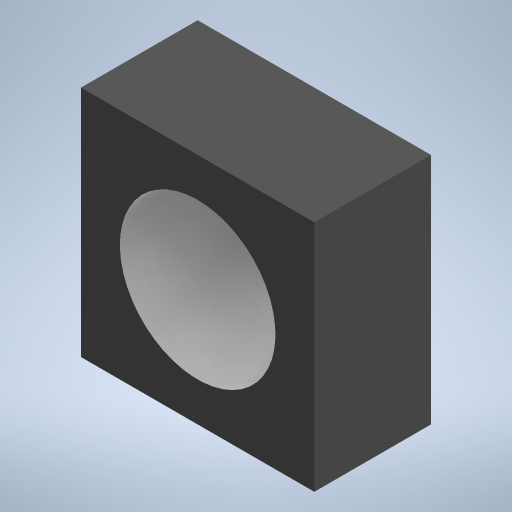
# Autodesk Inventor part: inge
Saved by Autodesk Inventor 2023.2 (Build 272271030, 271C)
## iProperties
Created: 2023-07-19
Part Number: inge
Material: Generic
Document SubType Name: Modeling
Designer: Cris Pat
Density: 1 g/cm^3
Appearance: Generic
Author: Cris Pat
Autodesk Inventor part; units mm, degrees
ref_plane "YZ Plane" through (0, 0, 0) normal (1, 0, 0) x (0, 1, 0)
ref_plane "XZ Plane" through (0, 0, 0) normal (0, 1, 0) x (-1, 0, 0)
ref_plane "XY Plane" through (0, 0, 0) normal (0, 0, 1) x (1, 0, 0)
sketch "Sketch1" plane through (0, 0, 0) normal (0, 0, 1) x (1, 0, 0)
  arc A0 (0, 50) -> (0, -50) centre (0, 0) ccw
  line L0 (0, -70) -> (0, 70) projected
  dimension "d0" = 100
  constraints: 2 point on circle, 2 point on line, 1 centre point, 1 coincident
  measures "d0" diameter of A0
revolve "Revolution1" add sketch "Sketch1" angle 360 about axis through (0, -10, 0) along (0, 1, 0)
sketch "Sketch2" plane through (0, 0, 0) normal (0, 0, 1) x (1, 0, 0)
  line L0 (-75, -75) -> (75, -75)
  line L1 (75, -75) -> (75, 75)
  line L2 (75, 75) -> (-75, 75)
  line L3 (-75, 75) -> (-75, -75)
  line L4 (-75, -75) -> (75, 75) construction
  line L5 (75, -75) -> (-75, 75) construction
  point P0 (0, 0)
  dimension "d2" = 150
  dimension "d3" = 150
  constraints: 12 end point, 2 midpoint, 2 parallel, 1 horizontal, 1 perpendicular
  measures "d2" distance of L2.end L1.end
  measures "d3" distance of L1.end L0.end
extrude "Extrusion1" add sketch "Sketch2" along normal mid plane 150 separate body
combine bodies "Combine1" operation type subtract main body 2 bodies to subtract 1
split body "Split1" result two bodies by plane through (0, 0, 0) normal (0, 0, 1) bodies 2 first body at (25, -25, 74.5)
body "Solid3"
body "Solid4"
